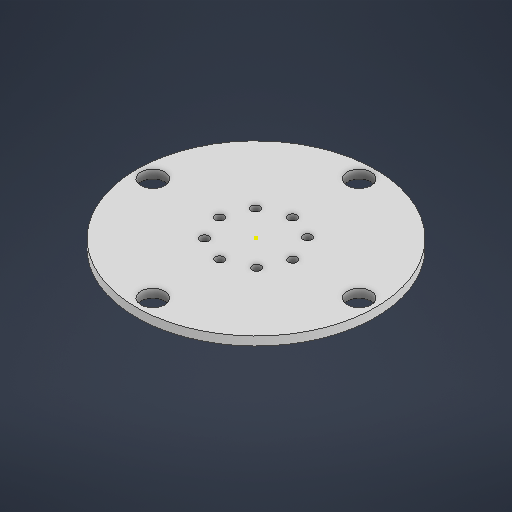
# Autodesk Inventor part: placa para pellet
Saved by Autodesk Inventor 2026.1 (Build 301233020, 233B)
## iProperties
Created: 2025-12-04
Part Number: placa para pellet
Material: Genérico
Document SubType Name: Modeling
Designer: benja
Density: 1 g/cm^3
Appearance: Valor por defecto
Author: benja
Autodesk Inventor part; units mm, degrees
ref_plane "YZ Plane" through (0, 0, 0) normal (1, 0, 0) x (0, 1, 0)
ref_plane "XZ Plane" through (0, 0, 0) normal (0, 1, 0) x (-1, 0, 0)
ref_plane "XY Plane" through (0, 0, 0) normal (0, 0, 1) x (1, 0, 0)
sketch "Boceto1" plane through (0, 0, 0) normal (0, 1, 0) x (-1, 0, 0)
  circle A0 centre (0, 0) radius 27.5
  dimension "d0" = 55
  constraints: 1 centre point, 1 coincident
  measures "d0" diameter of A0
extrude "Extrusión1" add sketch "Boceto1" along normal blind 2
sketch "Boceto6" plane through (0, 2, 0) normal (0, 1, 0) x (1, 0, 0)
  circle A0 centre (0, 0) radius 9.6625
  circle A1 centre (-8.777, -8.777) radius 2.75 projected
  circle A2 centre (0, 0) radius 7.1625
  circle A3 centre (8.4584, 0) radius 1
  circle A4 centre (0, -8.3447) radius 1
  circle A5 centre (0, 8.3727) radius 1
  circle A6 centre (-8.3635, 0) radius 1
  circle A7 centre (5.9357, -5.7822) radius 1
  circle A8 centre (-6.027, 5.9234) radius 1
  circle A9 centre (5.6693, 6.1791) radius 1
  circle A10 centre (-5.9197, -5.9092) radius 1
  dimension "d32" = 14.325
  dimension "d33" = 2
  dimension "d34" = 2
  dimension "d35" = 2
  dimension "d36" = 2
  dimension "d37" = 2
  dimension "d38" = 2
  dimension "d39" = 2
  dimension "d40" = 2
  constraints: 10 centre point, 2 coincident, 1 tangent
  measures "d32" diameter of A2
  measures "d33" diameter of A3
  measures "d34" diameter of A4
  measures "d35" diameter of A5
  measures "d36" diameter of A6
  measures "d37" diameter of A7
  measures "d38" diameter of A8
  measures "d39" diameter of A9
  measures "d40" diameter of A10
extrude "Extrusión3" cut sketch "Boceto6" against normal blind 50 contours A3 | A4 | A5 | A6 | A7 | A8 | A9 | A10
sketch "Boceto7" plane through (0, 0, 0) normal (0, 0, 1) x (1, 0, 0)
  line L0 (0, 0) -> (-7.1625, 0)
  line L1 (-11.527, 0) -> (-11.527, 2) projected
  line L2 (0, 0) -> (0, -5)
  line L3 (0, -5) -> (-7.1625, 0)
  dimension "d43" = 7.1625
  dimension "d44" = 5
  constraints: 6 end point, 1 perpendicular, 1 vertical
  measures "d43" distance of L0.start L0.end
  measures "d44" distance of L0.start L2.end
revolve "Revolución2" add sketch "Boceto7" angle 360 about axis through (0, 0, 0) along (0, -1, 0)
sketch "Boceto8" plane through (0, 2, 0) normal (0, 1, 0) x (1, 0, 0)
  circle A0 centre (0, 0) radius 7.1625 projected
  line L0 (0, 0) -> (0, 23.75)
  line L1 (0, 0) -> (23.75, 0)
  line L2 (0, 0) -> (0, -23.75)
  line L3 (0, 0) -> (-23.75, 0)
  circle A1 centre (-23.75, 0) radius 2.75
  circle A2 centre (0, 23.75) radius 2.75
  circle A3 centre (23.75, 0) radius 2.75
  circle A4 centre (0, -23.75) radius 2.75
  point P0 (0, 0)
  dimension "d57" = 23.75
  dimension "d58" = 23.75
  dimension "d59" = 23.75
  dimension "d60" = 23.75
  dimension "d61" = 5.5
  dimension "d62" = 5.5
  dimension "d63" = 5.5
  dimension "d64" = 5.5
  constraints: 8 end point, 4 centre point, 4 coincident, 2 horizontal, 2 vertical
  measures "d57" distance of L0.start L0.end
  measures "d58" distance of L0.start L1.end
  measures "d59" distance of L0.start L2.end
  measures "d60" distance of L0.start L3.end
  measures "d61" diameter of A1
  measures "d62" diameter of A2
  measures "d63" diameter of A3
  measures "d64" diameter of A4
extrude "Extrusión4" cut sketch "Boceto8" against normal blind 2 contours A4 | A1 | A2 | A3
sketch "Boceto10" plane through (0, 2, 0) normal (0, 1, 0) x (1, 0, 0)
  point P0 (0, 0)
